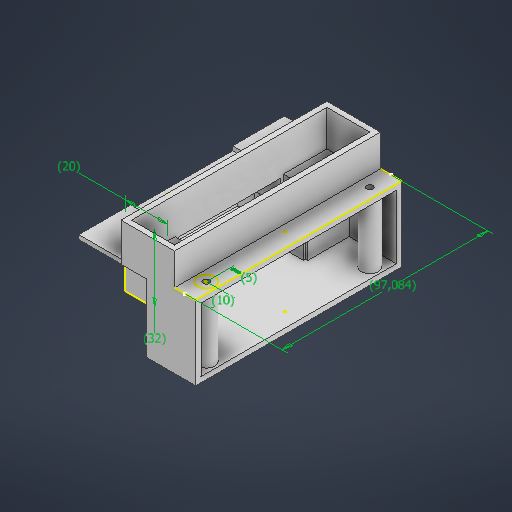
# Autodesk Inventor part: Sr. Batata
Saved by Autodesk Inventor 2026.1 (Build 301233020, 233B)
## iProperties
Created: 2025-11-07
Part Number: Sr. Batata
Material: Genérico
Document SubType Name: Modeling
Designer: david
Density: 1 g/cm^3
Appearance: Padrão
Author: david
Autodesk Inventor part; units mm, degrees
ref_plane "YZ Plane" through (0, 0, 0) normal (1, 0, 0) x (0, 1, 0)
ref_plane "XZ Plane" through (0, 0, 0) normal (0, 1, 0) x (-1, 0, 0)
ref_plane "XY Plane" through (0, 0, 0) normal (0, 0, 1) x (1, 0, 0)
sketch "Esboço1" plane through (0, 0, 0) normal (0, 1, 0) x (-1, 0, 0)
  line L0 (50, 50) -> (-50, 50)
  line L1 (-50, 50) -> (-50, -50)
  line L2 (-50, -50) -> (50, -50)
  line L3 (50, -50) -> (50, 50)
  line L4 (50, 50) -> (-50, -50) construction
  line L5 (-50, 50) -> (50, -50) construction
  line L6 (48.54211, 48.54211) -> (-6.685359, 48.54211)
  line L7 (-6.685359, 48.54211) -> (-6.685359, -48.542)
  line L8 (-6.685359, -48.542) -> (48.54211, -48.542)
  line L9 (48.54211, -48.542) -> (48.54211, 48.54211)
  line L10 (-6.685359, 48.54211) -> (3.314641, 48.54211)
  line L11 (3.314641, 48.54211) -> (3.314642, -48.542)
  line L12 (-1.685359, 48.54211) -> (8.314641, 48.54211)
  line L13 (-6.685359, 48.54211) -> (-1.685359, 48.54211)
  line L14 (-1.685359, 48.54211) -> (-1.685359, 38.54211)
  line L15 (-1.685359, 48.54211) -> (8.314641, 48.54211) construction
  circle A0 centre (-1.685359, 38.54211) radius 1.5
  line L16 (-6.685359, -48.542) -> (-1.685359, -48.542)
  line L17 (-1.685359, -48.542) -> (-1.685359, -38.542)
  circle A1 centre (-1.685359, -38.542) radius 1.5
  line L18 (48.54211, 0.000055) -> (28.54211, 0.000055)
  line L19 (28.54211, 48.54211) -> (28.54211, 26.54211)
  line L20 (28.54211, 26.54211) -> (48.54211, 26.54211)
  line L21 (28.54211, -48.542) -> (28.54211, -26.542)
  line L22 (28.54211, -48.542) -> (50.54211, -48.542) construction
  line L23 (28.54211, -26.542) -> (48.54211, -26.542)
  line L24 (28.54211, 26.54211) -> (28.54211, -26.542)
  point P0 (0, 0)
  dimension "d0" = 100
  dimension "d1" = 100
  dimension "d2" = 1.45789
  dimension "d3" = 1.458
  dimension "d4" = 43.31464
  dimension "d5" = 97.08411
  dimension "d6" = 10
  dimension "d7" = 10
  dimension "d8" = 5
  dimension "d9" = 10
  dimension "d10" = 90
  dimension "d11" = 3
  dimension "d12" = 5
  dimension "d13" = 10
  dimension "d14" = 90
  dimension "d15" = 3
  dimension "d16" = 55.22747
  dimension "d17" = 20
  dimension "d18" = 22
  dimension "d19" = 22
  dimension "d20" = 90
  dimension "d21" = 26.54205
  constraints: 50 end point, 10 point on line, 9 perpendicular, 6 horizontal, 4 midpoint, 4 parallel, 2 centre point, 2 coincident, 2 vertical, 1 collinear
  measures "d0" distance of L2.end L1.end
  measures "d1" distance of L1.end L0.end
  measures "d2" distance between parallel lines of L6 L0
  measures "d3" distance between parallel lines of L2 L8
  measures "d4" distance between parallel lines of L1 L7
  measures "d5" distance between parallel lines of L8 L6
  measures "d6" distance of L6.end L10.end
  measures "d7" distance of L12.start L12.end
  measures "d8" distance of L6.end L12.start
  measures "d9" distance of L12.start L14.end
  measures "d10" angle of L14 L15
  measures "d11" diameter of A0
  measures "d12" distance of L7.end L16.end
  measures "d13" distance of L16.end L17.end
  measures "d14" angle of L17 L16
  measures "d15" diameter of A1
  measures "d16" distance between parallel lines of L7 L9
  measures "d17" distance of L18.start L18.end
  measures "d18" distance of L19.start L19.end
  measures "d19" distance of L21.start L21.end
  measures "d20" angle of L22 L21
  measures "d21" distance of L18.end L19.end
sketch "Esboço1 outline for Extrusão1" plane through (0, 0, 0) normal (0, 1, 0) x (-1, 0, 0)
  line L0 (28.54211, -26.542) -> (28.54211, 26.54211)
  line L1 (28.54211, -48.542) -> (28.54211, -26.542)
  line L2 (3.314642, -48.542) -> (28.54211, -48.542)
  line L3 (3.314641, 48.54211) -> (3.314642, -48.542)
  line L4 (28.54211, 48.54211) -> (3.314641, 48.54211)
  line L5 (28.54211, 26.54211) -> (28.54211, 48.54211)
extrude "Extrusão1" add sketch "Esboço1 outline for Extrusão1" along normal blind 50
sketch "Esboço1 outline for Extrusão2" plane through (0, 0, 0) normal (0, 1, 0) x (-1, 0, 0)
  line L0 (3.314641, 48.54211) -> (-6.685359, 48.54211)
  line L1 (3.314642, -48.542) -> (3.314641, 48.54211)
  line L2 (-6.685359, 48.54211) -> (-6.685359, -48.542)
  line L3 (-6.685359, -48.542) -> (3.314642, -48.542)
  circle A0 centre (-1.685359, -38.542) radius 1.5
  circle A1 centre (-1.685359, 38.54211) radius 1.5
extrude "Extrusão2" add sketch "Esboço1 outline for Extrusão2" along normal blind 35
sketch "Esboço1 outline for Extrusão3" plane through (0, 0, 0) normal (0, 1, 0) x (-1, 0, 0)
  line L0 (28.54211, 26.54211) -> (28.54211, -26.542)
  line L1 (48.54211, 26.54211) -> (28.54211, 26.54211)
  line L2 (48.54211, -26.542) -> (48.54211, 26.54211)
  line L3 (28.54211, -26.542) -> (48.54211, -26.542)
extrude "Extrusão3" add sketch "Esboço1 outline for Extrusão3" along normal blind 32
thread "Rosca1" size "M3x0.5" class "6H" standard "ANSI Metric M Profile" length 20
thread "Rosca2" size "M3x0.5" class "6H" standard "ANSI Metric M Profile" length 20
shell "Casca1" thickness 2.5 removed faces 3 at (-35.208776, 32, -8.847297) at (-20.132954, 50, 16.18074) at (6.685359, 11.666667, 16.18074)
sketch "Esboço2" plane through (0, 35, 0) normal (0, 1, 0) x (1, 0, 0)
  line L0 (-3.314641, -48.54211) -> (6.685359, -48.54211)
  line L1 (6.685359, 48.542) -> (-3.314642, 48.542)
  point P0 (0, 0)
  point P1 (1.685359, -48.54211)
  point P2 (1.685358, 48.542)
  dimension "d33" = 97.08411
  constraints: 2 midpoint
  measures "d33" distance of point (1.685, -48.542) point (1.685, 48.542)
sketch "Esboço3" plane through (0, 35, 0) normal (0, 1, 0) x (1, 0, 0)
  point P0 (0, 0)
sketch "Esboço4" plane through (0, 35, 0) normal (0, 1, 0) x (1, 0, 0)
  circle A0 centre (1.685359, -38.54211) radius 4
  line L0 (-3.314641, -48.54211) -> (6.685359, -48.54211)
  line L1 (6.685359, -48.54211) -> (6.685359, 48.542)
  point P0 (0, 0)
  point P1 (1.685359, -48.54211)
  dimension "d34" = 10
  dimension "d35" = 5
  constraints: 1 midpoint
  measures "d34" distance of A0.centre point (1.685, -48.542)
  measures "d35" distance from line of L1 A0.centre
sketch "Esboço5" plane through (-26.04211, 2.5, 46.04211) normal (0, 1, 0) x (1, 0, 0)
  point P0 (26.04211, 46.04211)
sketch "Esboço6" plane through (-48.54211, 0, 26.54211) normal (0, 0, 1) x (1, 0, 0)
  point P0 (48.54211, 0)
sketch "Esboço7" plane through (-48.54211, 0, 26.54211) normal (0, 0, 1) x (1, 0, 0)
  line L0 (0, 0) -> (0, 32) projected
  line L1 (20, 0) -> (20, 50) projected
  point P0 (48.54211, 0)
  dimension "d36" = 20
  measures "d36" distance between parallel lines of L0 L1
sketch "Esboço8" plane through (-28.54211, 0, 48.54211) normal (-1, 0, 0) x (0, 0, 1)
  point P0 (-48.54211, 0)
sketch "Esboço9" plane through (-28.54211, 0, 48.54211) normal (-1, 0, 0) x (0, 0, 1)
  line L0 (-24.5, 32) -> (-22, 32)
  line L1 (0, 0) -> (-22, 0)
  line L2 (-22, 0) -> (-22, 32)
  line L3 (-22, 32) -> (0, 32)
  line L4 (0, 32) -> (0, 0)
  line L5 (-97.08411, 0) -> (-97.08411, 50)
  line L6 (-75.08411, 0) -> (-75.08411, 32)
  line L7 (-97.08411, 0) -> (-75.08411, 0)
  line L8 (-75.08411, 0) -> (-75.08411, 32)
  line L9 (-75.08411, 32) -> (-97.08411, 32)
  line L10 (-97.08411, 32) -> (-97.08411, 0)
  point P0 (-48.54211, 0)
  constraints: 16 end point, 4 parallel, 2 horizontal, 2 perpendicular
sketch "Esboço9 outline for Extrusão4" plane through (-28.54211, 0, 48.54211) normal (-1, 0, 0) x (0, 0, 1)
  line L0 (-22, 32) -> (-22, 0)
  line L1 (0, 32) -> (-22, 32)
  line L2 (0, 0) -> (0, 32)
  line L3 (-22, 0) -> (0, 0)
  line L4 (-97.08411, 0) -> (-75.08411, 0)
  line L5 (-97.08411, 32) -> (-97.08411, 0)
  line L6 (-75.08411, 32) -> (-97.08411, 32)
  line L7 (-75.08411, 0) -> (-75.08411, 32)
extrude "Extrusão4" cut sketch "Esboço9 outline for Extrusão4" against normal blind 12
sketch "Esboço10" plane through (-48.54211, 0, 26.54211) normal (0, 0, 1) x (1, 0, 0)
  line L0 (32, 0) -> (0, 0) projected
  line L1 (0, 32) -> (20, 32) projected
  point P0 (48.54211, 0)
  dimension "d39" = 32
  measures "d39" distance between parallel lines of L0 L1
sketch "Esboço11" plane through (0, 32, 0) normal (0, 1, 0) x (1, 0, 0)
  line L0 (-48.54211, 26.542) -> (-48.54211, -26.54211)
  line L1 (-16.54211, 48.542) -> (-28.54211, 48.542)
  line L2 (-48.54211, 24.069012) -> (-28.54211, 24.069012)
  line L3 (-28.54211, 24.069012) -> (-28.54211, 48.542)
  line L4 (-28.54211, 48.542) -> (-48.54211, 48.542)
  line L5 (-48.54211, 48.542) -> (-48.54211, 24.069012)
  line L6 (-48.54211, -24.04211) -> (-28.54211, -24.04211)
  line L7 (-28.54211, -24.04211) -> (-28.54211, -48.414968)
  line L8 (-28.54211, -48.414968) -> (-48.54211, -48.414968)
  line L9 (-48.54211, -48.414968) -> (-48.54211, -24.04211)
  point P0 (0, 0)
  point P1 (-48.54211, -26.54211)
  constraints: 16 end point, 4 parallel, 3 point on line, 2 horizontal, 2 perpendicular
sketch "Esboço11 outline for Extrusão5" plane through (0, 32, 0) normal (0, 1, 0) x (1, 0, 0)
  line L0 (-48.54211, -48.414968) -> (-28.54211, -48.414968)
  line L1 (-28.54211, -48.414968) -> (-28.54211, -24.04211)
  line L2 (-28.54211, -24.04211) -> (-48.54211, -24.04211)
  line L3 (-48.54211, -24.04211) -> (-48.54211, -48.414968)
  line L4 (-28.54211, 48.542) -> (-48.54211, 48.542)
  line L5 (-48.54211, 48.542) -> (-48.54211, 24.069012)
  line L6 (-48.54211, 24.069012) -> (-28.54211, 24.069012)
  line L7 (-28.54211, 24.069012) -> (-28.54211, 48.542)
extrude "Extrusão5" add sketch "Esboço11 outline for Extrusão5" along normal blind 2
sketch "Esboço12" plane through (-16.54211, 0, -26.542) normal (0, 0, -1) x (-1, 0, 0)
  line L0 (0, 0) -> (0, 32) projected
  line L1 (9.5, 2.5) -> (0, 2.5)
  line L2 (0, 2.5) -> (0, 32)
  line L3 (0, 32) -> (9.5, 32)
  line L4 (9.5, 32) -> (9.5, 2.5)
  point P0 (-16.54211, 0)
  point P1 (0, 2.5)
  constraints: 8 end point, 2 parallel, 1 horizontal, 1 perpendicular
sketch "Esboço12 outline for Extrusão6" plane through (-16.54211, 0, -26.542) normal (0, 0, -1) x (-1, 0, 0)
  line L0 (9.5, 2.5) -> (9.5, 32)
  line L1 (0, 2.5) -> (9.5, 2.5)
  line L2 (0, 32) -> (0, 2.5)
  line L3 (9.5, 32) -> (0, 32)
extrude "Extrusão6" add sketch "Esboço12 outline for Extrusão6" against normal blind 1
sketch "Esboço13" plane through (-16.54211, 0, 48.54211) normal (-1, 0, 0) x (0, 0, 1)
  line L0 (-97.08411, 0) -> (-97.08411, 32)
  line L1 (-75.08411, 2.5) -> (-75.08411, 0)
  line L2 (-97.08411, 32) -> (-75.08411, 32)
  line L3 (-75.08411, 32) -> (-75.08411, 2.5)
  line L4 (-75.08411, 2.5) -> (-97.08411, 2.5)
  line L5 (-97.08411, 2.5) -> (-97.08411, 32)
  point P0 (-48.54211, 0)
  constraints: 8 end point, 2 parallel, 1 horizontal, 1 perpendicular
sketch "Esboço13 outline for Extrusão7" plane through (-16.54211, 0, 48.54211) normal (-1, 0, 0) x (0, 0, 1)
  line L0 (-75.08411, 2.5) -> (-75.08411, 32)
  line L1 (-97.08411, 2.5) -> (-75.08411, 2.5)
  line L2 (-97.08411, 32) -> (-97.08411, 2.5)
  line L3 (-75.08411, 32) -> (-97.08411, 32)
extrude "Extrusão7" add sketch "Esboço13 outline for Extrusão7" against normal blind 1
sketch "Esboço14" plane through (-16.54211, 32, -26.542) normal (0, 1, 0) x (1, 0, 0)
  line L0 (0, 0) -> (0, -1) projected
  line L1 (-9.5, 0) -> (-9.5, 19.5) projected
  line L2 (0, -1) -> (-9.5, -1)
  line L3 (-9.5, -1) -> (-9.5, 19.5)
  line L4 (-9.5, 19.5) -> (0, 19.5)
  line L5 (0, 19.5) -> (0, -1)
  point P0 (16.54211, -26.542)
  constraints: 8 end point, 2 parallel, 1 horizontal, 1 perpendicular
sketch "Esboço14 outline for Extrusão8" plane through (-16.54211, 32, -26.542) normal (0, 1, 0) x (1, 0, 0)
  line L0 (-9.5, -1) -> (0, -1)
  line L1 (-9.5, 0) -> (-9.5, -1)
  line L2 (-9.5, 19.5) -> (-9.5, 0)
  line L3 (0, 19.5) -> (-9.5, 19.5)
  line L4 (0, 0) -> (0, 19.5)
  line L5 (0, -1) -> (0, 0)
extrude "Extrusão8" add sketch "Esboço14 outline for Extrusão8" along normal blind 1
sketch "Esboço15" plane through (-48.54211, 0, 26.54211) normal (0, 0, 1) x (1, 0, 0)
  line L0 (22.5, 2.5) -> (22.5, 33) projected
  line L1 (22.5, 2.5) -> (32, 2.5)
  line L2 (32, 2.5) -> (32, 32)
  line L3 (32, 32) -> (22.5, 32)
  line L4 (22.5, 32) -> (22.5, 2.5)
  point P0 (48.54211, 0)
  point P1 (22.5, 32)
  constraints: 8 end point, 2 parallel, 1 horizontal, 1 perpendicular
sketch "Esboço15 outline for Extrusão9" plane through (-48.54211, 0, 26.54211) normal (0, 0, 1) x (1, 0, 0)
  line L0 (32, 2.5) -> (32, 32)
  line L1 (22.5, 2.5) -> (32, 2.5)
  line L2 (22.5, 32) -> (22.5, 2.5)
  line L3 (32, 32) -> (22.5, 32)
extrude "Extrusão9" add sketch "Esboço15 outline for Extrusão9" against normal blind 1
sketch "Esboço16" plane through (-16.54211, 0, 48.54211) normal (-1, 0, 0) x (0, 0, 1)
  line L0 (-22, 0) -> (-22, 32) projected
  line L1 (-22, 2.5) -> (-2.5, 2.5) projected
  line L2 (-22, 32) -> (-2.5, 32)
  line L3 (-2.5, 32) -> (-2.5, 2.5)
  line L4 (-2.5, 2.5) -> (-22, 2.5)
  line L5 (-22, 2.5) -> (-22, 32)
  point P0 (-48.54211, 0)
  constraints: 8 end point, 2 parallel, 1 horizontal, 1 perpendicular
sketch "Esboço16 outline for Extrusão10" plane through (-16.54211, 0, 48.54211) normal (-1, 0, 0) x (0, 0, 1)
  line L0 (-2.5, 2.5) -> (-2.5, 32)
  line L1 (-22, 2.5) -> (-2.5, 2.5)
  line L2 (-22, 32) -> (-22, 2.5)
  line L3 (-2.5, 32) -> (-22, 32)
extrude "Extrusão10" add sketch "Esboço16 outline for Extrusão10" against normal blind 1
sketch "Esboço17" plane through (-16.54211, 32, 46.04211) normal (0, 1, 0) x (1, 0, 0)
  line L0 (0, 20.5) -> (0, 19.5) projected
  line L1 (0, 0) -> (-9.5, 0) projected
  line L2 (0, 20.5) -> (-9.5, 20.5)
  line L3 (-9.5, 20.5) -> (-9.5, 0)
  line L4 (-9.5, 0) -> (0, 0)
  line L5 (0, 0) -> (0, 20.5)
  point P0 (16.54211, 46.04211)
  point P1 (0, 19.5)
  constraints: 8 end point, 2 parallel, 1 horizontal, 1 perpendicular
sketch "Esboço17 outline for Extrusão11" plane through (-16.54211, 32, 46.04211) normal (0, 1, 0) x (1, 0, 0)
  line L0 (-9.5, 20.5) -> (-9.5, 0)
  line L1 (0, 20.5) -> (-9.5, 20.5)
  line L2 (0, 19.5) -> (0, 20.5)
  line L3 (0, 0) -> (0, 19.5)
  line L4 (-9.5, 0) -> (0, 0)
extrude "Extrusão11" add sketch "Esboço17 outline for Extrusão11" along normal blind 1
sketch "Esboço18" plane through (-16.54211, 0, -26.542) normal (0, 0, -1) x (-1, 0, 0)
  line L0 (32, 0) -> (32, 32) projected
  line L1 (0, 0) -> (0, 32) projected
  line L2 (0, 32) -> (0, 0) projected
  line L3 (0, 0) -> (0, 15.8)
  line L4 (0, 15.8) -> (15.8, 15.8)
  line L5 (9.8, 20.8) -> (21.8, 20.8)
  line L6 (21.8, 20.8) -> (21.8, 10.8)
  line L7 (21.8, 10.8) -> (9.8, 10.8)
  line L8 (9.8, 10.8) -> (9.8, 20.8)
  line L9 (9.8, 20.8) -> (21.8, 10.8) construction
  line L10 (21.8, 20.8) -> (9.8, 10.8) construction
  point P0 (-16.54211, 0)
  dimension "d54" = 32
  dimension "d55" = 15.8
  dimension "d56" = 15.8
  dimension "d57" = 12
  dimension "d58" = 10
  constraints: 16 end point, 2 midpoint, 2 parallel, 2 perpendicular, 1 horizontal, 1 point on line
  measures "d54" distance between parallel lines of L0 L1
  measures "d55" distance of L1.start L3.end
  measures "d56" distance of L3.end L4.end
  measures "d57" distance of L6.end L7.end
  measures "d58" distance of L5.end L6.end
sketch "Esboço18 outline for Extrusão12" plane through (-16.54211, 0, -26.542) normal (0, 0, -1) x (-1, 0, 0)
  line L0 (9.8, 10.8) -> (21.8, 10.8)
  line L1 (9.8, 20.8) -> (9.8, 10.8)
  line L2 (21.8, 20.8) -> (9.8, 20.8)
  line L3 (21.8, 10.8) -> (21.8, 20.8)
extrude "Extrusão12" cut sketch "Esboço18 outline for Extrusão12" against normal blind 2.5
sketch "Esboço19" plane through (-48.54211, 0, 26.54211) normal (0, 0, 1) x (1, 0, 0)
  line L0 (32, 2.5) -> (32, 0) projected
  line L1 (32, 0) -> (32, 15.8)
  line L2 (32, 32) -> (32, 2.5) projected
  line L3 (32, 0) -> (47.8, 0) construction
  line L4 (32, 15.8) -> (16.2, 15.8)
  line L5 (22.2, 10.8) -> (10.2, 10.8)
  line L6 (10.2, 10.8) -> (10.2, 20.8)
  line L7 (10.2, 20.8) -> (22.2, 20.8)
  line L8 (22.2, 20.8) -> (22.2, 10.8)
  line L9 (22.2, 10.8) -> (10.2, 20.8) construction
  line L10 (10.2, 10.8) -> (22.2, 20.8) construction
  point P0 (48.54211, 0)
  dimension "d61" = 15.8
  dimension "d62" = 90
  dimension "d63" = 15.8
  dimension "d64" = 90
  dimension "d65" = 12
  dimension "d66" = 10
  constraints: 18 end point, 3 perpendicular, 2 horizontal, 2 midpoint, 2 parallel, 1 collinear
  measures "d61" distance of L0.end L1.end
  measures "d62" angle of L3 L1
  measures "d63" distance of L1.end L4.end
  measures "d64" angle of L4 L1
  measures "d65" distance of L6.end L7.end
  measures "d66" distance of L5.end L6.end
sketch "Esboço19 outline for Extrusão13" plane through (-48.54211, 0, 26.54211) normal (0, 0, 1) x (1, 0, 0)
  line L0 (22.2, 20.8) -> (10.2, 20.8)
  line L1 (22.2, 10.8) -> (22.2, 20.8)
  line L2 (10.2, 10.8) -> (22.2, 10.8)
  line L3 (10.2, 20.8) -> (10.2, 10.8)
extrude "Extrusão13" cut sketch "Esboço19 outline for Extrusão13" against normal blind 2.5
sketch "Esboço20" plane through (-46.04211, 2.5, -24.042) normal (0, 1, 0) x (1, 0, 0)
  line L0 (7.7, 2.5) -> (7.7, 0)
  line L1 (0, -48.08411) -> (20, -48.08411)
  line L2 (7.7, 0) -> (20, 0)
  line L3 (20, 0) -> (20, -48.08411)
  line L4 (20, -48.08411) -> (7.7, -48.08411)
  line L5 (7.7, -48.08411) -> (7.7, 0)
  point P0 (46.04211, -24.042)
  point P1 (7.7, -48.08411)
  constraints: 8 end point, 2 parallel, 1 horizontal, 1 perpendicular
sketch "Esboço20 outline for Extrusão14" plane through (-46.04211, 2.5, -24.042) normal (0, 1, 0) x (1, 0, 0)
  line L0 (20, -48.08411) -> (20, 0)
  line L1 (7.7, -48.08411) -> (20, -48.08411)
  line L2 (7.7, 0) -> (7.7, -48.08411)
  line L3 (20, 0) -> (7.7, 0)
extrude "Extrusão14" add sketch "Esboço20 outline for Extrusão14" along normal blind 8.3
sketch "Esboço21" plane through (-46.04211, 2.5, 24.04211) normal (0, 1, 0) x (1, 0, 0)
  line L0 (0, 48.08411) -> (0, 0)
  line L1 (19.7, 0) -> (7.7, 0)
  line L2 (0, 48.08411) -> (7.7, 48.08411)
  line L3 (7.7, 48.08411) -> (7.7, 0)
  line L4 (7.7, 0) -> (0, 0)
  line L5 (0, 0) -> (0, 48.08411)
  point P0 (46.04211, 24.04211)
  constraints: 8 end point, 2 parallel, 1 horizontal, 1 perpendicular
sketch "Esboço21 outline for Extrusão15" plane through (-46.04211, 2.5, 24.04211) normal (0, 1, 0) x (1, 0, 0)
  line L0 (0, 0) -> (7.7, 0)
  line L1 (0, 48.08411) -> (0, 0)
  line L2 (7.7, 48.08411) -> (0, 48.08411)
  line L3 (7.7, 0) -> (7.7, 48.08411)
extrude "Extrusão15" add sketch "Esboço21 outline for Extrusão15" along normal blind 8.3
